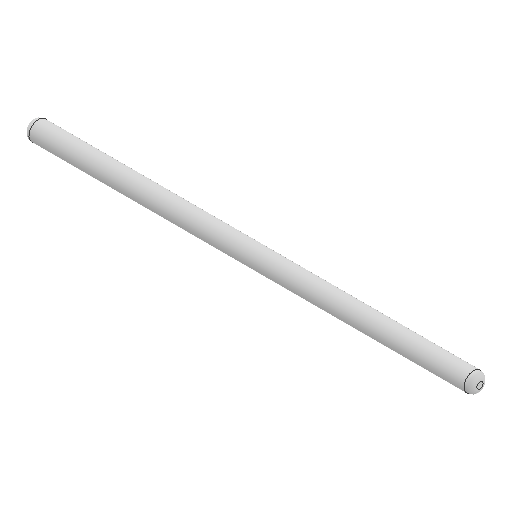
# Autodesk Inventor part: Шпилька скрепления деталей
Saved by Autodesk Inventor 2022 (Build 260153000, 153)
## iProperties
Created: 2023-02-19
Part Number: Шпилька скрепления деталей
Material: Типовые
Document SubType Name: Modeling
Designer: Глеб
Density: 1 g/cm^3
Appearance: По умолчанию
Author: Глеб
Autodesk Inventor part; units mm, degrees
ref_plane "YZ Plane" through (0, 0, 0) normal (1, 0, 0) x (0, 1, 0)
ref_plane "XZ Plane" through (0, 0, 0) normal (0, 1, 0) x (-1, 0, 0)
ref_plane "XY Plane" through (0, 0, 0) normal (0, 0, 1) x (1, 0, 0)
sketch "Эскиз1" plane through (0, 0, 0) normal (1, 0, 0) x (0, 1, 0)
  circle A0 centre (0, 0) radius 1.5
  dimension "d0" = 3
  constraints: 1 centre point, 1 coincident
  measures "d0" diameter of A0
extrude "Выдавливание1" add sketch "Эскиз1" along normal mid plane 70
fillet "Сопряжение1" radius 1 2 edges at (-35, -1.5, 0) (35, -1.5, 0)
